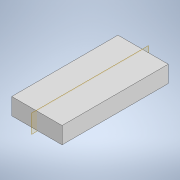
# Autodesk Inventor part: ESC
Saved by Autodesk Inventor 2021 (Build 250183000, 183)
## iProperties
Created: 2020-11-24
Part Number: ESC
Material: Generic
Document SubType Name: Modeling
Designer: Kanenas
Mass: 9 g
Surface Area: 20.4 cm^2
Volume: 4.104 cm^3
Density: 2.19298 g/cm^3
Appearance: Default
Author: Kanenas
Autodesk Inventor part; units mm, degrees
ref_plane "XZ Plane" through (0, 0, 0) normal (0, 1, 0) x (-1, 0, 0)
ref_plane "XY Plane" through (0, 0, 0) normal (0, 0, 1) x (1, 0, 0)
sketch "Sketch1" plane through (0, 0, 0) normal (0, 0, 1) x (1, 0, 0)
  line L0 (-9, 3) -> (9, 3)
  line L1 (9, 3) -> (9, -3)
  line L2 (9, -3) -> (-9, -3)
  line L3 (-9, -3) -> (-9, 3)
  line L4 (-9, 3) -> (9, -3) construction
  line L5 (9, 3) -> (-9, -3) construction
  point P0 (0, 0)
  dimension "d0" = 18
  dimension "d1" = 6
  constraints: 12 end point, 2 midpoint, 2 parallel, 1 horizontal, 1 perpendicular
  measures "d0" distance of L0.start L0.end
  measures "d1" distance of L0.end L1.end
extrude "Extrusion1" add sketch "Sketch1" along normal blind 38
body "Solid1"
